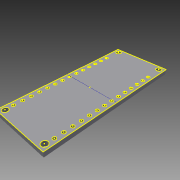
# Autodesk Inventor part: Arduino Nano
Saved by Autodesk Inventor 2015 (Build 190159000, 159)
## iProperties
Created: 2018-12-22
Part Number: Arduino Nano
Material: Типовые
Document SubType Name: Modeling
Designer: kostya
Density: 1 g/cm^3
Appearance: По умолчанию
Author: kostya
Autodesk Inventor part; units mm, degrees
ref_plane "YZ Plane" through (0, 0, 0) normal (1, 0, 0) x (0, 1, 0)
ref_plane "XZ Plane" through (0, 0, 0) normal (0, 1, 0) x (-1, 0, 0)
ref_plane "XY Plane" through (0, 0, 0) normal (0, 0, 1) x (1, 0, 0)
sketch "Эскиз1" plane through (0, 0, 0) normal (0, 0, 1) x (1, 0, 0)
  line L0 (8.9, 21.6) -> (-8.9, 21.6)
  line L1 (-8.9, 21.6) -> (-8.9, -21.6)
  line L2 (-8.9, -21.6) -> (8.9, -21.6)
  line L3 (8.9, -21.6) -> (8.9, 21.6)
  line L4 (8.9, 21.6) -> (-8.9, -21.6) construction
  line L5 (-8.9, 21.6) -> (8.9, -21.6) construction
  line L6 (8.9, 21.6) -> (7.4, 21.6) construction
  line L7 (8.9, 21.6) -> (8.9, 20.1) construction
  line L8 (7.4, 21.6) -> (8.9, 21.6) construction
  line L9 (8.9, 21.6) -> (8.9, 20.1) construction
  line L10 (8.9, 20.1) -> (7.4, 20.1) construction
  line L11 (7.4, 20.1) -> (7.4, 21.6) construction
  circle A0 centre (7.4, 20.1) radius 0.9
  line L12 (-8.9, 0) -> (8.9, 0) construction
  line L13 (0, 21.6) -> (0, -21.6) construction
  line L14 (-8.9, 20.1) -> (-7.4, 20.1) construction
  line L15 (-7.4, 20.1) -> (-7.4, 21.6) construction
  circle A1 centre (-7.4, 20.1) radius 0.9
  line L16 (8.9, -20.1) -> (7.4, -20.1) construction
  line L17 (7.4, -20.1) -> (7.4, -21.6) construction
  circle A2 centre (7.4, -20.1) radius 0.9
  circle A3 centre (-7.4, -20.1) radius 0.9
  line L18 (-8.9, -20.1) -> (-7.4, -20.1) construction
  line L19 (-7.6, 21.6) -> (7.6, 21.6) construction
  line L20 (7.6, 21.6) -> (7.6, -21.6) construction
  line L21 (7.6, -21.6) -> (-7.6, -21.6) construction
  line L22 (-7.6, -21.6) -> (-7.6, 21.6) construction
  line L23 (-7.6, 21.6) -> (7.6, -21.6) construction
  line L24 (7.6, 21.6) -> (-7.6, -21.6) construction
  line L25 (-7.6, -21.6) -> (-7.6, -17.8) construction
  circle A4 centre (-7.6, -17.8) radius 0.5
  circle A5 centre (-7.6, -15.3) radius 0.5
  circle A6 centre (-7.6, -12.8) radius 0.5
  circle A7 centre (-7.6, -10.3) radius 0.5
  circle A8 centre (-7.6, -7.8) radius 0.5
  circle A9 centre (-7.6, -5.3) radius 0.5
  circle A10 centre (-7.6, -2.8) radius 0.5
  circle A11 centre (-7.6, -0.3) radius 0.5
  circle A12 centre (-7.6, 2.2) radius 0.5
  circle A13 centre (-7.6, 4.7) radius 0.5
  circle A14 centre (-7.6, 7.2) radius 0.5
  circle A15 centre (-7.6, 9.7) radius 0.5
  circle A16 centre (-7.6, 12.2) radius 0.5
  circle A17 centre (-7.6, 14.7) radius 0.5
  line L26 (8.9, 0) -> (-8.9, 0) construction
  line L27 (7.6, -21.6) -> (7.6, 21.6) construction
  circle A18 centre (7.6, -17.8) radius 0.5
  circle A19 centre (7.6, -15.3) radius 0.5
  circle A20 centre (7.6, -12.8) radius 0.5
  circle A21 centre (7.6, -10.3) radius 0.5
  circle A22 centre (7.6, -7.8) radius 0.5
  circle A23 centre (7.6, -5.3) radius 0.5
  circle A24 centre (7.6, -2.8) radius 0.5
  circle A25 centre (7.6, -0.3) radius 0.5
  circle A26 centre (7.6, 2.2) radius 0.5
  circle A27 centre (7.6, 4.7) radius 0.5
  circle A28 centre (7.6, 7.2) radius 0.5
  circle A29 centre (7.6, 9.7) radius 0.5
  circle A30 centre (7.6, 12.2) radius 0.5
  circle A31 centre (7.6, 14.7) radius 0.5
  point P0 (0, 0)
  dimension "d0" = 17.8
  dimension "d1" = 43.2
  dimension "d2" = 1.5
  dimension "d3" = 1.5
  dimension "d4" = 1.8
  dimension "d5" = 15.2
  dimension "d6" = 3.8
  dimension "d7" = 1
  dimension "d10" = 2.5
  constraints: 56 end point, 38 symmetric about line, 32 centre point, 29 coincident, 8 midpoint, 6 parallel, 5 point on line, 3 horizontal, 3 perpendicular, 1 vertical, 56 other
  measures "d0" distance of L2.end L1.end
  measures "d1" distance of L1.end L0.end
  measures "d2" distance of L0.start L6.end
  measures "d3" distance of L0.start L7.end
  measures "d4" diameter of A0
  measures "d5" distance of L20.end L21.end
  measures "d6" distance of L21.end L25.end
  measures "d7" diameter of A4
  measures "d10" distance of A4.centre A5.centre
extrude "Выдавливание1" add sketch "Эскиз1" along normal blind 1.6
sketch "Эскиз2" plane through (0, 0, 1.6) normal (0, 0, 1) x (1, 0, 0)
  circle A0 centre (7.4, -20.1) radius 0.9 projected
  circle A1 centre (-7.4, -20.1) radius 0.9 projected
  circle A2 centre (-7.4, 20.1) radius 0.9 projected
  circle A3 centre (7.4, 20.1) radius 0.9 projected
  circle A4 centre (7.6, 12.2) radius 0.5 projected
  circle A5 centre (7.6, 14.7) radius 0.5 projected
  circle A6 centre (7.6, 9.7) radius 0.5 projected
  circle A7 centre (7.6, 7.2) radius 0.5 projected
  circle A8 centre (7.6, 4.7) radius 0.5 projected
  circle A9 centre (7.6, 2.2) radius 0.5 projected
  circle A10 centre (7.6, -0.3) radius 0.5 projected
  circle A11 centre (7.6, -2.8) radius 0.5 projected
  circle A12 centre (7.6, -5.3) radius 0.5 projected
  circle A13 centre (7.6, -7.8) radius 0.5 projected
  circle A14 centre (7.6, -12.8) radius 0.5 projected
  circle A15 centre (7.6, -10.3) radius 0.5 projected
  circle A16 centre (7.6, -15.3) radius 0.5 projected
  circle A17 centre (7.6, -17.8) radius 0.5 projected
  circle A18 centre (-7.6, 14.7) radius 0.5 projected
  circle A19 centre (-7.6, 12.2) radius 0.5 projected
  circle A20 centre (-7.6, 9.7) radius 0.5 projected
  circle A21 centre (-7.6, 7.2) radius 0.5 projected
  circle A22 centre (-7.6, 4.7) radius 0.5 projected
  circle A23 centre (-7.6, 2.2) radius 0.5 projected
  circle A24 centre (-7.6, -0.3) radius 0.5 projected
  circle A25 centre (-7.6, -2.8) radius 0.5 projected
  circle A26 centre (-7.6, -5.3) radius 0.5 projected
  circle A27 centre (-7.6, -7.8) radius 0.5 projected
  circle A28 centre (-7.6, -10.3) radius 0.5 projected
  circle A29 centre (-7.6, -12.8) radius 0.5 projected
  circle A30 centre (-7.6, -15.3) radius 0.5 projected
  circle A31 centre (-7.6, -17.8) radius 0.5 projected
  line L0 (8.9, 21.6) -> (-8.9, 21.6) projected
  line L1 (-8.9, 21.6) -> (-8.9, -21.6) projected
  line L2 (-8.9, -21.6) -> (8.9, -21.6) projected
  line L3 (8.9, -21.6) -> (8.9, 21.6) projected
  line L4 (-8.9, 21.6) -> (-8.9, -21.6) construction
  line L5 (-8.9, 0) -> (8.9, 0) construction
  point P0 (0, 0)
  constraints: 2 end point, 2 midpoint
